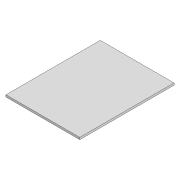
# Autodesk Inventor part: Placeholder_tray
Saved by Autodesk Inventor 2022 (Build 260153000, 153)
## iProperties
Created: 2022-10-27
Part Number: Placeholder_tray
Material: Generic
Document SubType Name: Modeling
Designer: MVeszpremi
Density: 1 g/cm^3
Appearance: Default
Author: MVeszpremi
Autodesk Inventor part; units mm, degrees
ref_plane "YZ Plane" through (0, 0, 0) normal (1, 0, 0) x (0, 1, 0)
ref_plane "XZ Plane" through (0, 0, 0) normal (0, 1, 0) x (-1, 0, 0)
ref_plane "XY Plane" through (0, 0, 0) normal (0, 0, 1) x (1, 0, 0)
sketch "Sketch1" plane through (0, 0, 0) normal (0, 1, 0) x (-1, 0, 0)
  line L0 (175, 225) -> (-175, 225)
  line L1 (-175, 225) -> (-175, -225)
  line L2 (-175, -225) -> (175, -225)
  line L3 (175, -225) -> (175, 225)
  line L4 (175, 225) -> (-175, -225) construction
  line L5 (-175, 225) -> (175, -225) construction
  point P0 (0, 0)
  dimension "d0" = 450
  dimension "d1" = 350
  constraints: 12 end point, 2 midpoint, 2 parallel, 1 horizontal, 1 perpendicular
  measures "d0" distance of L2.end L0.start
  measures "d1" distance of L1.end L2.end
extrude "Extrusion1" add sketch "Sketch1" along normal blind 4
sketch "Sketch2" plane through (0, 4, 0) normal (0, 1, 0) x (1, 0, 0)
  line L0 (-180, -230) -> (180, -230)
  line L1 (180, -230) -> (180, 230)
  line L2 (180, 230) -> (-180, 230)
  line L3 (-180, 230) -> (-180, -230)
  line L4 (-180, -230) -> (180, 230) construction
  line L5 (180, -230) -> (-180, 230) construction
  line L6 (-175, 225) -> (-175, -225) projected
  line L7 (-175, -225) -> (175, -225) projected
  line L8 (175, -225) -> (175, 225) projected
  line L9 (175, 225) -> (-175, 225) projected
  line L10 (-175, 225) -> (-175, -225) projected
  line L11 (-175, -225) -> (175, -225) projected
  point P0 (0, 0)
  dimension "d4" = 5
  dimension "d5" = 5
  constraints: 12 end point, 2 midpoint, 2 parallel, 1 horizontal, 1 perpendicular
  measures "d4" distance between parallel lines of L3 L6
  measures "d5" distance between parallel lines of L7 L0
extrude "Extrusion2" add sketch "Sketch2" against normal blind 10
body "Solid1"
